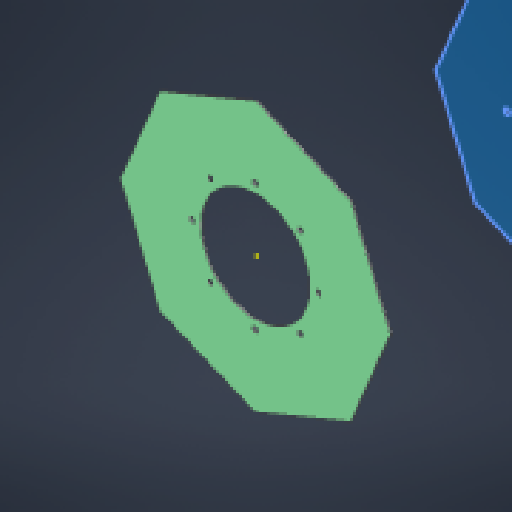
# Autodesk Inventor part: DMF 01 21 Барабан торец НОС v2.1
Saved by Autodesk Inventor 2026.2 (Build 302298010, 298A)
## iProperties
Created: 2024-04-28
Part Number: DMF 01 21 Барабан торец НОС v2.1
Material: Generic
Document SubType Name: Sheet Metal
Designer: pokla
Density: 1 g/cm^3
Appearance: Default
Sheet Metal Rule: Default
Flat Pattern Width: 57 cm
Flat Pattern Length: 57 cm
Flat Pattern Area: 3249 cm^2
Sheet Metal Width: 570,000 mm
Sheet Metal Length: 570,000 mm
Sheet Metal Area: 324900,000 mm^2
Stock Number: Барабан_Торец_Нос
Author: pokla
Autodesk Inventor part; units mm, degrees
ref_plane "YZ Plane" through (0, 0, 0) normal (1, 0, 0) x (0, 1, 0)
ref_plane "XZ Plane" through (0, 0, 0) normal (0, 1, 0) x (-1, 0, 0)
ref_plane "XY Plane" through (0, 0, 0) normal (0, 0, 1) x (1, 0, 0)
sketch "Sketch2" plane through (0, 0, 0) normal (0, 0, 1) x (1, 0, 0)
  line L0 (-218.1296, 218.1296) -> (0, 308.4818)
  line L1 (0, 308.4818) -> (218.1296, 218.1296)
  line L2 (218.1296, 218.1296) -> (308.4818, 0)
  line L3 (308.4818, 0) -> (218.1296, -218.1296)
  line L4 (218.1296, -218.1296) -> (0, -308.4818)
  line L5 (0, -308.4818) -> (-218.1296, -218.1296)
  line L6 (-218.1296, -218.1296) -> (-308.4818, 0)
  line L7 (-308.4818, 0) -> (-218.1296, 218.1296)
  circle A0 centre (0, 0) radius 125
  dimension "d23" = 570
  dimension "d26" = 250
  measures "d23" distance between parallel lines of L6 L2
  measures "d26" diameter of A0
extrude "Plate1" add sketch "Sketch2" against normal blind 3
sketch "Sketch4" plane through (0, 0, 0) normal (0, 0, 1) x (1, 0, 0)
  circle A0 centre (0, 145) radius 6.25
  circle A1 centre (0, 0) radius 125 projected
  dimension "d16" = 12.5
  dimension "d17" = 145
  constraints: 1 centre point, 1 vertical alignment
  measures "d16" diameter of A0
  measures "d17" distance of point (0, 0) A0.centre
extrude "Extrusion1" cut sketch "Sketch4" against normal up to surface (3 mm away) contours A0
pattern_circular "Circular Pattern1" count 8 over 360 about axis through (0, 0, -10) along (0, 0, 1) of "Extrusion1"
sketch "Sketch6" plane through (0, 0, 0) normal (0, 0, 1) x (1, 0, 0)
  line L0 (202.8222, 202.8222) -> (286.8339, 0)
  line L1 (286.8339, 0) -> (202.8222, -202.8222)
  line L2 (202.8222, -202.8222) -> (0, -286.8339)
  line L3 (0, -286.8339) -> (-202.8222, -202.8222)
  line L4 (-202.8222, -202.8222) -> (-286.8339, 0)
  line L5 (-286.8339, 0) -> (-202.8222, 202.8222)
  line L6 (-202.8222, 202.8222) -> (0, 286.8339)
  line L7 (0, 286.8339) -> (202.8222, 202.8222)
  point P0 (0, 0)
  point P1 (0, 0)
  dimension "d27" = 530
  constraints: 16 end point, 1 coincident, 1 vertical alignment, 17 other
  measures "d27" distance between parallel lines of L3 L7
mark "Mark1"
equation "\"d26\" = Вал_ось_диаметр_НОС"
equation "\"d27\" = Барабан_размер_по_плоскостям"
equation "\"d15\" = Thickness"
equation "\"BendRadius\" = Thickness"
equation "\"BendReliefWidth\" = Thickness"
equation "\"BendReliefDepth\" = 0.5 * Thickness"
equation "\"CornerReliefSize\" = 4 * Thickness"
equation "\"MinimumRemnant\" = 2 * Thickness"
equation "\"TransitionRadius\" = BendRadius"
equation "\"JacobiRadiusSize\" = BendRadius"
equation "\"GapSize\" = Thickness"
equation "\"Вал_ось_диаметр_НОС\" = 250"
equation "\"Барабан_размер_по_плоскостям\" = 530"
equation "\"Thickness\" = 3"
body "Solid1"
